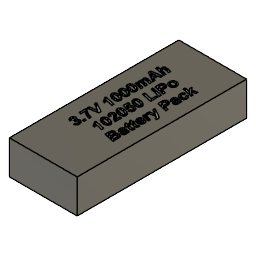
Battery (Autodesk Fusion 360 design; units mm, degrees)
part number: 2026-06-18-10-40-38-082
Autodesk Fusion 360 part; units mm, degrees
sketch "Sketch1" plane through (0, 0, 0) normal (0, 0, 1) x (1, 0, 0)
  line L0 (-60, 60) -> (-40, 60)
  line L1 (-40, 60) -> (-40, 10)
  line L2 (-40, 10) -> (-60, 10)
  line L3 (-60, 10) -> (-60, 60)
  dimension "d1" = 50
  dimension "d2" = 20
  constraint horizontal L0
  constraint vertical L1
  constraint horizontal L2
  constraint vertical L3
  measures "d1" distance of L0.start L2.end
  measures "d2" distance of L0.start L0.end
extrude "Extrude1" add sketch "Sketch1" along normal blind 10
sketch "Sketch2" plane through (0, 0, 10) normal (0, 0, 1) x (-1, 0, 0)
  line L0 (60, -10) -> (40, -10)
  line L1 (40, -10) -> (40, -60)
  line L2 (40, -60) -> (60, -60)
  line L3 (60, -60) -> (60, -10)
  line L4 (45, -20) -> (45, -54) construction
  line L5 (45, -54) -> (55, -54) construction
  line L6 (55, -54) -> (55, -20) construction
  line L7 (55, -20) -> (45, -20) construction
  dimension "d5" = 3
  dimension "d6" = 0
  text T0 "3.7V 1000mAh 102050 LiPo Battery Pack" font "Arial" height 3 bold italic align centre middle in box 34 x 10 at (45, -20) x (0, -1) y (1, 0) spacing 1
extrude "Extrude2" cut sketch "Sketch2" against normal blind 2 text T0
equation "d6 = '3.7V 1000mAh 102050 LiPo Battery Pack'"
